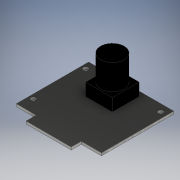
# Autodesk Inventor part: Pixy Sketch
Saved by Autodesk Inventor 2018 (Build 220112000, 112)
## iProperties
Created: 2018-08-30
Part Number: Pixy Sketch
Material: Generic
Document SubType Name: Modeling
Designer: matth
Density: 1 g/cm^3
Appearance: Default
Author: matth
Autodesk Inventor part; units mm, degrees
ref_plane "YZ Plane" through (0, 0, 0) normal (1, 0, 0) x (0, 1, 0)
ref_plane "XZ Plane" through (0, 0, 0) normal (0, 1, 0) x (-1, 0, 0)
ref_plane "XY Plane" through (0, 0, 0) normal (0, 0, 1) x (1, 0, 0)
sketch "Sketch1" plane through (0, 0, 0) normal (0, 0, 1) x (1, 0, 0)
  line L0 (0, 0) -> (0, 8.5)
  line L1 (0, 8.5) -> (8.5, 8.5)
  line L2 (8.5, 8.5) -> (8.5, -8.5)
  line L3 (8.5, -8.5) -> (-8.5, -8.5)
  line L4 (-8.5, -8.5) -> (-8.5, 8.5)
  line L5 (-8.5, 8.5) -> (0, 8.5)
  line L6 (0, 8.5) -> (0, 10.25)
  line L7 (0, 10.25) -> (-23.8, 10.25)
  line L8 (-23.8, 10.25) -> (-23.8, 6.92)
  circle A0 centre (-23.8, 6.92) radius 1.5
  line L9 (0, 10.25) -> (23.8, 10.25)
  line L10 (23.8, 10.25) -> (23.8, 6.92)
  circle A1 centre (23.8, 6.92) radius 1.5
  line L11 (-23.8, 6.92) -> (-23.8, -26.28)
  circle A2 centre (-23.8, -26.28) radius 1.5
  line L12 (0, 0) -> (0, 6.92)
  line L13 (-25.3, 6.92) -> (-26.55, 6.92)
  line L14 (-26.55, 6.92) -> (-26.55, -28.83)
  line L15 (-26.55, 6.92) -> (-26.55, 11.5)
  line L16 (-26.55, 11.5) -> (27.45, 11.5)
  line L17 (27.45, 11.5) -> (27.45, 11.5)
  line L18 (27.45, 11.5) -> (27.45, -28.83)
  line L19 (27.45, -28.83) -> (-26.55, -28.83)
  dimension "d8" = 3
  dimension "d0" = 8.5
  dimension "d1" = 8.5
  dimension "d2" = 17
  dimension "d3" = 17
  dimension "d4" = 17
  dimension "d5" = 1.75
  dimension "d6" = 23.8
  dimension "d7" = 3.33
  dimension "d9" = 23.8
  dimension "d10" = 3.33
  dimension "d11" = 3
  dimension "d12" = 33.2
  dimension "d13" = 3
  dimension "d14" = 1.25
  dimension "d15" = 35.75
  dimension "d16" = 4.58
  dimension "d17" = 0
  dimension "d33" = 54
  constraints: 40 end point, 10 perpendicular, 4 point on line, 4 vertical, 3 coincident, 2 centre point, 2 horizontal, 1 horizontal alignment, 2 other
  measures "d0" distance of L0.start L0.end
  measures "d1" distance of L0.end L1.end
  measures "d2" distance of L1.end L2.end
  measures "d3" distance of L2.end L3.end
  measures "d4" distance of L3.end L4.end
  measures "d5" distance of L0.end L6.end
  measures "d6" distance of L6.end L7.end
  measures "d7" distance of L7.end L8.end
  measures "d9" distance of L6.end L9.end
  measures "d10" distance of L9.end L10.end
  measures "d11" diameter of A1
  measures "d12" distance of L11.start L11.end
  measures "d13" diameter of A2
  measures "d14" distance of L13.start L13.end
  measures "d15" distance of L13.end L14.end
  measures "d16" distance of L13.end L15.end
  measures "d17" distance of L16.end L17.end
  measures "d33" distance of L15.end L16.end
extrude "Extrusion1" add sketch "Sketch1" along normal blind 1.65
sketch "Sketch2" plane through (0, 0, 1.65) normal (0, 0, 1) x (1, 0, 0)
  line L0 (-8.5, 8.5) -> (-8.5, -8.5) projected
  line L1 (8.5, 8.5) -> (8.5, -8.5) projected
  line L2 (-8.5, 8.5) -> (8.5, 8.5)
  line L3 (8.5, 8.5) -> (8.5, -8.5)
  line L4 (8.5, -8.5) -> (-8.5, -8.5)
  line L5 (-8.5, -8.5) -> (-8.5, 8.5)
  point P0 (0, 0)
  constraints: 8 end point, 2 parallel, 1 horizontal, 1 perpendicular
extrude "Extrusion2" add sketch "Sketch2" along normal blind 8 and the other way blind 1.65
sketch "Sketch3" plane through (0, 0, 9.65) normal (0, 0, 1) x (1, 0, 0)
  circle A0 centre (0, 0) radius 7.5
  dimension "d24" = 15
  constraints: 1 centre point, 1 coincident
  measures "d24" diameter of A0
extrude "Extrusion3" add sketch "Sketch3" along normal blind 16
sketch "Sketch4" plane through (0, 0, 1.65) normal (0, 0, 1) x (1, 0, 0)
  line L0 (-26.55, -28.83) -> (27.45, -28.83) projected
  line L1 (-26.55, -28.83) -> (27.45, -28.83)
  line L2 (27.45, -28.83) -> (27.45, -34.38)
  line L3 (27.45, -34.38) -> (-26.55, -34.38)
  line L4 (-26.55, -34.38) -> (-26.55, -28.83)
  point P0 (0, 0)
  dimension "d27" = 5.55
  dimension "d34" = 54
  constraints: 8 end point, 2 parallel, 1 horizontal, 1 perpendicular
  measures "d27" distance of L1.end L2.end
  measures "d34" distance of L2.end L3.end
extrude "Extrusion4" add sketch "Sketch4" against normal blind 1.65
sketch "Sketch5" plane through (0, 0, 1.65) normal (0, 0, 1) x (1, 0, 0)
  line L0 (27.45, -34.38) -> (-26.55, -34.38) projected
  line L1 (-26.55, -34.38) -> (-13.95, -34.38)
  line L2 (-13.95, -34.38) -> (-13.95, -40.78)
  line L3 (-13.95, -40.78) -> (14.65, -40.78)
  line L4 (14.65, -40.78) -> (14.65, -34.38)
  line L5 (14.65, -34.38) -> (-13.95, -34.38)
  point P0 (0, 0)
  dimension "d30" = 12.6
  dimension "d31" = 6.4
  dimension "d32" = 28.6
  constraints: 10 end point, 2 perpendicular, 2 point on line, 1 collinear, 1 vertical
  measures "d30" distance of L0.end L1.end
  measures "d31" distance of L1.end L2.end
  measures "d32" distance of L2.end L3.end
extrude "Extrusion5" add sketch "Sketch5" against normal blind 1.65
equation "\"d9\" = d6"
body "Solid1"
